Autodesk Inventor part; units mm, degrees
(part 2 of 2)
  point P14 (28.5, 17)
  point P15 (25, 12)
  point P16 (78.5, 17)
  point P17 (75, 12)
  point P18 (128.5, 17)
  point P19 (125, 12)
  point P20 (101.5834, -33.4298)
  point P21 (101.5834, 33.4298)
  point P22 (-2.6725, 99.5864)
  point P23 (-4.1682, 100.7298)
  point P24 (-2.6725, -97.3136)
  point P25 (-2.6725, -100.4136)
  dimension "d160" = 50
  dimension "d163" = 24
  dimension "d166" = 7
  dimension "d167" = 10
  dimension "d168" = 25
  dimension "d169" = 7
  dimension "d172" = 50
  dimension "d175" = 24
  dimension "d178" = 18
  dimension "d179" = 15
  dimension "d182" = 8
  dimension "d185" = 360
  dimension "d189" = 10
  dimension "d190" = 0
  dimension "d191" = 20
  dimension "d192" = 40
  dimension "d193" = 3.1
  dimension "d196" = 50
  dimension "d199" = 50
  constraints: 154 end point, 41 centre point, 16 point on circle, 12 tangent, 11 symmetric about line, 9 horizontal, 9 midpoint, 9 point on line, 7 parallel, 6 vertical, 3 equal radius, 3 perpendicular, 1 collinear, 162 other
  measures "d160" distance of L2.end L6.start
  measures "d163" distance of L2.end L14.start
  measures "d166" distance of L28.end L27.end
  measures "d167" distance of L27.end L26.end
  measures "d168" distance from line of L5 point (25, -12)
  measures "d169" distance from line of L4 point (28.5, -7)
  measures "d172" distance of L27.end L32.start
  measures "d175" distance of L27.end L40.start
  measures "d178" diameter of A3
  measures "d179" distance edge to line of A0 L54
  measures "d182" diameter of A6
  measures "d189" radius of A14
  measures "d190" distance between parallel lines of L194 L195
  measures "d191" distance of L196.start L196.end
  measures "d192" distance of L198.end L196.start
  measures "d193" diameter of A156
  measures "d196" distance of A156.centre A157.centre
  measures "d199" distance of A156.centre A161.centre
extrude "Выдавливание10" cut sketch "Эскиз16" against normal blind 10
